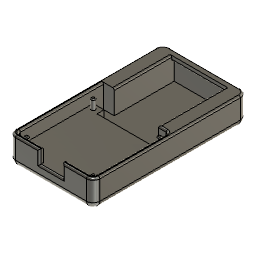
case (Autodesk Fusion 360 design; units mm, degrees)
Autodesk Fusion 360 part; units mm, degrees
other "Base Mesh Feature1"
sketch "Sketch1" plane through (0, 0, 0) normal (0, 0, 1) x (1, 0, 0) in component "PCB"
  line L0 (-21.0951, 22.3314) -> (20.9049, 22.3314)
  line L1 (22.4049, 20.8314) -> (22.4049, -21.1686)
  line L2 (20.9049, -22.6686) -> (-21.0951, -22.6686)
  line L3 (-22.5951, -21.1686) -> (-22.5951, 20.8314)
  circle A0 centre (19.9049, 19.8314) radius 1.5
  circle A1 centre (-20.0951, 19.8314) radius 1.5
  circle A2 centre (-20.0951, -20.1686) radius 1.5
  circle A3 centre (19.9049, -20.1686) radius 1.5
  line L4 (-0.0951, 22.3314) -> (-0.0951, 20.3314)
  line L5 (10.0649, 21.6014) -> (-10.2551, 21.6014)
  line L6 (-10.2551, 21.6014) -> (-10.2551, 19.0614)
  line L7 (-10.2551, 19.0614) -> (10.0649, 19.0614)
  line L8 (10.0649, 19.0614) -> (10.0649, 21.6014)
  line L9 (10.0649, 21.6014) -> (-10.2551, 19.0614) construction
  line L10 (-10.2551, 21.6014) -> (10.0649, 19.0614) construction
  arc A4 (-21.0951, 22.3314) -> (-22.5951, 20.8314) centre (-21.0951, 20.8314) ccw
  arc A5 (-22.5951, -21.1686) -> (-21.0951, -22.6686) centre (-21.0951, -21.1686) ccw
  arc A6 (20.9049, -22.6686) -> (22.4049, -21.1686) centre (20.9049, -21.1686) ccw
  arc A7 (22.4049, 20.8314) -> (20.9049, 22.3314) centre (20.9049, 20.8314) ccw
  point P0 (22.4049, 22.3314)
  point P1 (22.4049, -22.6686)
  point P2 (-22.5951, -22.6686)
  point P3 (-0.0951, 20.3314)
  dimension "d1" = 45
  dimension "d2" = 45
  dimension "d3" = 3
  dimension "d4" = 2.5
  dimension "d5" = 2.5
  dimension "d6" = 3
  dimension "d7" = 2.5
  dimension "d8" = 2.5
  dimension "d9" = 3
  dimension "d10" = 2.5
  dimension "d11" = 2.5
  dimension "d12" = 3
  dimension "d13" = 2.5
  dimension "d14" = 2.5
  dimension "d15" = 2
  dimension "d16" = 20.32
  dimension "d17" = 2.54
  dimension "d18" = 1.5
  constraint horizontal L0
  constraint vertical L1
  constraint horizontal L2
  constraint vertical L3
  constraint perpendicular L0 L4
  constraint horizontal L5
  constraint perpendicular L5 L6
  constraint parallel L5 L7
  constraint parallel L6 L8
  constraint coincident L9 P3
  constraint coincident L10 P3
  constraint coincident P3 L4.end
  constraint coincident L0 L4.start
  constraint tangent L0 A4
  constraint tangent L3 A4
  constraint coincident P2 L2
  constraint coincident P2 L3
  constraint tangent L2 A5
  constraint tangent L3 A5
  constraint equal A4 A5
  constraint coincident P1 L1
  constraint coincident P1 L2
  constraint tangent L1 A6
  constraint tangent L2 A6
  constraint equal A4 A6
  constraint coincident P0 L0
  constraint coincident P0 L1
  constraint tangent L0 A7
  constraint tangent L1 A7
  constraint equal A4 A7
  measures "d1" distance of P0 P1
  measures "d2" distance of P1 P2
  measures "d3" diameter of A0
  measures "d4" distance of L1 A0.centre
  measures "d5" distance of L0 A0.centre
  measures "d6" diameter of A1
  measures "d7" distance of L0 A1.centre
  measures "d8" distance of L3 A1.centre
  measures "d9" diameter of A2
  measures "d10" distance of L2 A2.centre
  measures "d11" distance of L3 A2.centre
  measures "d12" diameter of A3
  measures "d13" distance of L1 A3.centre
  measures "d14" distance of L2 A3.centre
  measures "d15" distance of L4.start P3
  measures "d16" distance of L6.end L7.end
  measures "d17" distance of L5.end L6.end
  measures "d18" radius of A4
sketch "Sketch1 (2)" plane through (0, 0, 0) normal (0, 0, 1) x (1, 0, 0) in component "Screen"
  line L0 (10.0649, 21.6014) -> (-10.2551, 21.6014)
  line L1 (-10.2551, 19.0614) -> (10.0649, 19.0614)
  line L2 (-10.2551, 21.6014) -> (-10.2551, 19.0614)
  line L3 (10.0649, 19.0614) -> (10.0649, 21.6014)
  line L4 (-10.2551, 20.3314) -> (10.0649, 20.3314)
  line L5 (-16.0951, 18.8314) -> (15.9049, 18.8314)
  line L6 (-0.0951, 20.3314) -> (-0.0951, 18.8314) construction
  line L7 (-16.0951, 18.8314) -> (-16.0951, 62.5314)
  line L8 (-16.0951, 62.5314) -> (15.9049, 62.5314)
  line L9 (15.9049, 62.5314) -> (15.9049, 18.8314)
  circle A0 centre (-13.5951, 60.0314) radius 1
  circle A1 centre (13.4049, 60.0314) radius 1
  line L10 (-16.0951, 57.5514) -> (15.9049, 57.5514)
  line L11 (15.9049, 57.5514) -> (15.9049, 23.8314)
  line L12 (15.9049, 23.8314) -> (-16.0951, 23.8314)
  line L13 (-16.0951, 23.8314) -> (-16.0951, 57.5514)
  dimension "d19" = 32
  dimension "d20" = 1.5
  dimension "d21" = 43.7
  dimension "d22" = 32
  dimension "d23" = 2
  dimension "d24" = 2.5
  dimension "d25" = 2.5
  dimension "d26" = 2
  dimension "d27" = 2.5
  dimension "d28" = 2.5
  dimension "d29" = 33.72
  dimension "d30" = 5
  constraint midpoint L2 L4.start
  constraint midpoint L3 L4.end
  constraint horizontal L5
  constraint midpoint L4 L6.start
  constraint coincident L5 L6.end
  constraint perpendicular L5 L6
  constraint midpoint L5 L6.end
  constraint perpendicular L5 L7
  constraint perpendicular L7 L8
  constraint horizontal L10
  constraint vertical L11
  constraint horizontal L12
  constraint vertical L13
  constraint coincident L7 L10.start
  measures "d19" distance of L5.start L5.end
  measures "d20" distance of L4 L5
  measures "d21" distance of L5.start L7.end
  measures "d22" distance of L7.end L8.end
  measures "d23" diameter of A0
  measures "d24" distance of L8 A0.centre
  measures "d25" distance of L7 A0.centre
  measures "d26" diameter of A1
  measures "d27" distance of L9 A1.centre
  measures "d28" distance of L8 A1.centre
  measures "d29" distance of L10.start L12.end
  measures "d30" distance of L5 L12
sketch "Sketch3" plane through (0, 0, 0) normal (0, 0, 1) x (1, 0, 0) in component "Case"
  line L0 (15.9049, 57.5514) -> (15.9049, 23.8314)
  line L1 (15.9049, 62.5314) -> (15.9049, 18.8314)
  line L2 (-16.0951, 62.5314) -> (15.9049, 62.5314)
  line L3 (-16.0951, 18.8314) -> (-16.0951, 62.5314)
  line L4 (-22.5951, -21.1686) -> (-22.5951, 20.8314)
  line L5 (20.9049, -22.6686) -> (-21.0951, -22.6686)
  arc A0 (-22.5951, -21.1686) -> (-21.0951, -22.6686) centre (-21.0951, -21.1686) ccw
  arc A1 (-21.0951, 22.3314) -> (-22.5951, 20.8314) centre (-21.0951, 20.8314) ccw
  line L6 (-21.0951, 22.3314) -> (20.9049, 22.3314)
  circle A2 centre (-20.0951, 19.8314) radius 1.5
  arc A3 (22.4049, 20.8314) -> (20.9049, 22.3314) centre (20.9049, 20.8314) ccw
  line L7 (22.4049, 20.8314) -> (22.4049, -21.1686)
  arc A4 (20.9049, -22.6686) -> (22.4049, -21.1686) centre (20.9049, -21.1686) ccw
  circle A5 centre (19.9049, -20.1686) radius 1.5
  circle A6 centre (19.9049, 19.8314) radius 1.5
  circle A7 centre (-20.0951, -20.1686) radius 1.5
  line L8 (-16.0951, 18.8314) -> (15.9049, 18.8314)
  circle A8 centre (13.4049, 60.0314) radius 1
  circle A9 centre (-13.5951, 60.0314) radius 1
  arc A10 (-21.0951, 22.6814) -> (-22.9451, 20.8314) centre (-21.0951, 20.8314) ccw construction
  line L9 (-22.9451, -21.1686) -> (-22.9451, 20.8314)
  arc A11 (-22.9451, -21.1686) -> (-21.0951, -23.0186) centre (-21.0951, -21.1686) ccw
  line L10 (20.9049, -23.0186) -> (-21.0951, -23.0186)
  arc A12 (20.9049, -23.0186) -> (22.7549, -21.1686) centre (20.9049, -21.1686) ccw
  line L11 (22.7549, 20.8314) -> (22.7549, -21.1686)
  arc A13 (22.7549, 20.8314) -> (20.9049, 22.6814) centre (20.9049, 20.8314) ccw
  line L12 (-21.0951, 22.6814) -> (20.9049, 22.6814)
  circle A14 centre (-20.0951, 19.8314) radius 1.2
  circle A15 centre (19.9049, 19.8314) radius 1.2
  circle A16 centre (19.9049, -20.1686) radius 1.2
  circle A17 centre (-20.0951, -20.1686) radius 1.2
  line L13 (-25.4451, -25.5186) -> (25.2549, -25.5186)
  line L14 (25.2549, -25.5186) -> (25.2549, 67.0314)
  line L15 (25.2549, 67.0314) -> (-25.4451, 67.0314)
  line L16 (-25.4451, 67.0314) -> (-25.4451, -25.5186)
  circle A18 centre (-13.5951, 60.0314) radius 0.8
  circle A19 centre (13.4049, 60.0314) radius 0.8
  line L17 (-16.4451, 18.4814) -> (16.2549, 18.4814)
  line L18 (16.2549, 62.8814) -> (16.2549, 18.4814)
  line L19 (-16.4451, 62.8814) -> (16.2549, 62.8814)
  line L20 (-16.4451, 18.4814) -> (-16.4451, 62.8814)
  line L21 (-16.4451, 62.8814) -> (-16.4451, 64.8814)
  line L22 (-16.4451, 64.8814) -> (16.2549, 64.8814)
  line L23 (16.2549, 64.8814) -> (16.2549, 62.8814)
  line L24 (-22.9451, 20.8314) -> (-22.9451, 28.8314)
  line L25 (-22.9451, 28.8314) -> (-16.4451, 28.8314)
  line L26 (-21.0951, 22.6814) -> (-22.9451, 22.6814)
  dimension "d31" = -0.35
  dimension "d32" = -0.3
  dimension "d33" = -0.3
  dimension "d34" = -0.3
  dimension "d35" = -0.3
  dimension "d36" = 2.5
  dimension "d37" = 2.5
  dimension "d38" = 2.5
  dimension "d39" = 4.5
  dimension "d40" = -0.2
  dimension "d41" = -0.2
  dimension "d42" = -0.35
  dimension "d43" = 2
  dimension "d44" = 8
  constraint horizontal L13
  constraint vertical L14
  constraint horizontal L15
  constraint vertical L16
  constraint perpendicular L15 L21
  constraint perpendicular L21 L22
  constraint vertical L23
  constraint parallel L9 L24
  constraint coincident L20 L25.end
  constraint perpendicular L20 L25
  constraint coincident L24 L26.end
  constraint tangent A10 L26
  constraint perpendicular L24 L26
  measures "d36" distance of L10 L13
  measures "d37" distance of L11 L14
  measures "d38" distance of L9 L16
  measures "d39" distance of L2 L15
  measures "d43" distance of L19.start L21.end
  measures "d44" distance of A10.end L24.end
extrude "Extrude1" add sketch "Sketch3" along normal blind 14.2 contours L13 L14 L15 L16 makes body 1
extrude "Extrude2" add sketch "Sketch3" along normal blind 6.2 contours L4 L5 A0 A1 L6 A3 L7 A4 L9 A11 L10 A12 L11 A13 L12 L18 L20 L24 L26 | L4 L5 A0 A1 L6 A3 L7 A4 L17 L18 L20 | A2 | A5 | A6 | A7 | A14 | A15 | A16 | A17 bodies 1
extrude "Extrude3" add sketch "Sketch3" against normal blind 2.5 contours L0 L1 L2 L3 L12 L18 L19 L20 | L0 L1 L2 L3 L12 | L1 L3 L6 L12 | L1 L3 L6 L8 L17 L18 L20 | L1 L3 L6 L8 | L3 L6 L12 L20 | L4 L5 A0 A1 L6 A3 L7 A4 L9 A11 L10 A12 L11 A13 L12 L18 L20 L24 L26 | L4 L5 A0 A1 L6 A3 L7 A4 L17 L18 L20 | L12 L20 L24 L25 L26 | L19 L21 L22 L23 | A2 | A5 | A6 | A7 | A8 | A9 | A14 | A15 | A16 | A17 | L13 L14 L15 L16 | A18 | A19 bodies 1
copy_body "CutPasteBodies1" bodies 1 removing the originals makes body 2 in component "Case"
extrude "Extrude1'" add sketch "Sketch3" along normal blind 12 contours A14 | A15 | A16 | A17 bodies 2 in component "Case"
other "Modify1"
sketch "Sketch2" plane through (0, 0, 14.2) normal (0, 0, 1) x (-1, 0, 0)
  arc A0 (22.9451, 21.1686) -> (21.0951, 23.0186) centre (21.0951, 21.1686) ccw
  line L0 (22.9451, 21.1686) -> (22.9451, -28.8314)
  line L1 (22.9451, -28.8314) -> (16.4451, -28.8314)
  line L2 (16.4451, -28.8314) -> (16.4451, -64.8814)
  line L3 (16.4451, -64.8814) -> (-16.2549, -64.8814)
  line L4 (-16.2549, -64.8814) -> (-16.2549, -22.6814)
  line L5 (-16.2549, -22.6814) -> (-20.9049, -22.6814)
  arc A1 (-22.7549, -20.8314) -> (-20.9049, -22.6814) centre (-20.9049, -20.8314) ccw
  line L6 (-22.7549, -20.8314) -> (-22.7549, 21.1686)
  arc A2 (-20.9049, 23.0186) -> (-22.7549, 21.1686) centre (-20.9049, 21.1686) ccw
  line L7 (-20.9049, 23.0186) -> (21.0951, 23.0186)
  line L8 (25.4451, -67.0314) -> (25.4451, 25.5186)
  line L9 (25.4451, 25.5186) -> (-25.2549, 25.5186)
  line L10 (-25.2549, 25.5186) -> (-25.2549, -67.0314)
  line L11 (-25.2549, -67.0314) -> (25.4451, -67.0314)
  line L12 (25.4451, 25.5186) -> (-25.2549, 25.5186)
  line L13 (-20.9049, 23.0186) -> (21.0951, 23.0186)
  line L14 (7.0951, 23.0186) -> (7.0951, 25.5186)
  line L15 (-6.9049, 23.0186) -> (-6.9049, 25.5186)
  line L16 (0.0951, 25.5186) -> (0.0951, 23.0186) construction
  dimension "d53" = 7
  dimension "d54" = 7
  constraint coincident L7 L14.start
  constraint coincident L9 L14.end
  constraint perpendicular L9 L14
  constraint coincident L7 L15.start
  constraint coincident L12 L15.end
  constraint perpendicular L12 L15
  constraint midpoint L12 L16.start
  constraint midpoint L7 L16.end
  measures "d53" distance of L14 L16
  measures "d54" distance of L15 L16
extrude "Extrude2'" cut sketch "Sketch2" against normal blind 8 contours L7 L9 L12 L13 L14 L15 bodies 2 in component "Case"
sketch "Sketch3 (2)" plane through (0, 64.8814, 0) normal (0, -1, 0) x (1, 0, 0)
  line L0 (-16.4451, 0) -> (16.2549, 0)
  line L1 (16.2549, 0) -> (16.2549, 14.2)
  line L2 (16.2549, 14.2) -> (-16.4451, 14.2)
  line L3 (-16.4451, 14.2) -> (-16.4451, 0)
  line L4 (-16.4451, 14.2) -> (16.2549, 14.2)
  line L5 (-16.4451, 0) -> (-16.4451, 14.2)
  line L6 (16.2549, 0) -> (16.2549, 14.2)
  line L7 (-16.4451, 11.2) -> (16.2549, 11.2)
  dimension "d57" = 3
  constraint coincident L5 L7.start
  constraint coincident L6 L7.end
  constraint perpendicular L6 L7
  measures "d57" distance of L4 L7
extrude "Extrude3'" add sketch "Sketch3 (2)" along normal blind 1.5 contours L1 L2 L3 L4 L5 L6 L7 bodies 2 in component "Case"
fillet "Fillet1" radius 1 19 edges at (16.0799, -25.5186, 14.2) (25.2549, 20.7564, 14.2) (-16.2701, -25.5186, 14.2) (-25.4451, 20.7564, 14.2) (-14.0951, -23.0186, 14.2) (-22.4033, -22.4768, 14.2) (-22.9451, 3.8314, 14.2) (18.5799, 22.6814, 14.2) (22.213, 22.1395, 14.2) (22.7549, -0.1686, 14.2) (22.213, -22.4768, 14.2) (13.9049, -23.0186, 14.2) (-0.0951, 67.0314, 14.2) (-16.4451, 46.1064, 14.2) (-0.0951, 63.3814, 11.2) (16.2549, 43.0314, 14.2) (-0.0951, -25.5186, 6.2) (6.9049, -25.5186, 10.2) (-7.0951, -25.5186, 10.2) on bodies 2 in component "Case"
fillet "Fillet2" radius 4 12 edges at (25.2549, -25.5186, 5.35) (24.962, -25.2257, 13.9071) (-25.4451, -25.5186, 5.35) (-25.1522, -25.2257, 13.9071) (-25.1522, 66.7385, 13.9071) (-25.4451, 67.0314, 5.35) (25.2549, 67.0314, 5.35) (24.962, 66.7385, 13.9071) (25.2549, 20.7564, -2.5) (-0.0951, 67.0314, -2.5) (-25.4451, 20.7564, -2.5) (-0.0951, -25.5186, -2.5) on bodies 2 in component "Case"
extrude "Extrude4" add sketch "Sketch1 (2)" along normal blind 1.2 separate body contours L5 L7 L9 L12 | L7 L8 L9 L10 sketch seen with x (1, 0, 0) y (0, 1, 0) z (0, 0, 1) at (0, 0, 12) makes body 3 at (4.2831, 62.0084, 12) makes body 4 at (-14.1485, 21.4214, 12)
extrude "Extrude5" add sketch "Sketch1 (2)" along normal blind 3.7 contours L7 L9 L10 L11 L12 L13 sketch seen with x (1, 0, 0) y (0, 1, 0) z (0, 0, 1) at (0, 0, 12) bodies 3 4
copy_body "CutPasteBodies1'" bodies 3 body 3 seen with x (1, 0, 0) y (0, 1, 0) z (0, 0, 1) at (0, 0, -12) removing the originals makes body 5 in component "Screen"
fillet "Fillet3" radius 0.5 4 edges at (-21.2139, 19.3975, 12) (-21.2139, -20.6025, 12) (18.7861, 19.3975, 12) (18.7861, -20.6025, 12) on bodies 2 in component "Case"
component "PCB" placed x (1, 0, 0) y (0, 1, 0) z (0, 0, 1) at (0, 0, 0)
component "Case" placed x (1, 0, 0) y (0, 1, 0) z (0, 0, 1) at (0, 0, 0)
component "Screen" placed x (1, 0, 0) y (0, 1, 0) z (0, 0, 1) at (0, 0, 12)
